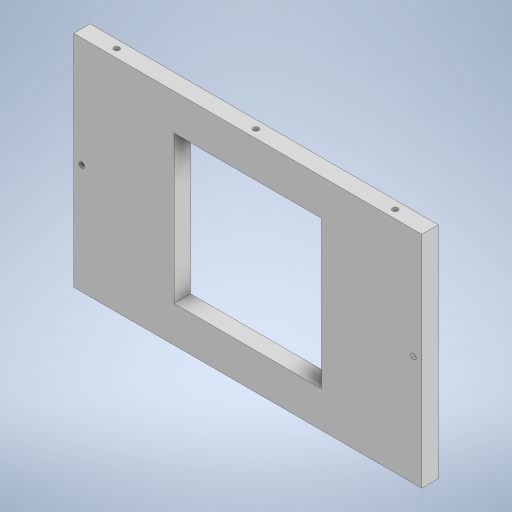
# Autodesk Inventor part: Lateral
Saved by Autodesk Inventor 2023.2 (Build 272271030, 271C)
## iProperties
Created: 2023-04-15
Part Number: Lateral
Material: Generic
Document SubType Name: Modeling
Designer: victo
Density: 1 g/cm^3
Appearance: Default
Author: victo
## iProperties of the stored document Lateral1-2_3DPrint.ipt
Created: 2023-05-16
Part Number: Lateral1-2_3DPrint
Material: Generic
Document SubType Name: Modeling
Designer: VICTOR
Density: 1 g/cm^3
Appearance: Default
Author: VICTOR
Autodesk Inventor part; units mm, degrees
ref_plane "YZ Plane" through (0, 0, 0) normal (1, 0, 0) x (0, 1, 0)
ref_plane "XZ Plane" through (0, 0, 0) normal (0, 1, 0) x (-1, 0, 0)
ref_plane "XY Plane" through (0, 0, 0) normal (0, 0, 1) x (1, 0, 0)
sketch "Sketch1" plane through (0, 0, 0) normal (0, 0, 1) x (1, 0, 0)
  line L0 (0, 0) -> (190, 0)
  line L1 (190, 0) -> (190, 120)
  line L2 (190, 120) -> (0, 120)
  line L3 (0, 120) -> (0, 0)
  dimension "d0" = 190
  dimension "d1" = 120
  constraints: 8 end point, 2 parallel, 1 horizontal, 1 perpendicular
  measures "d0" distance of L2.end L1.end
  measures "d1" distance of L1.end L0.end
extrude "Extrusion1" add sketch "Sketch1" along normal blind 9
sketch "Sketch2" plane through (0, 0, 9) normal (0, 0, 1) x (1, 0, 0)
  line L0 (190, 0) -> (190, 120) projected
  line L1 (190, 120) -> (0, 120) projected
  line L2 (0, 120) -> (0, 0) projected
  line L3 (0, 0) -> (190, 0) projected
  line L4 (135.25, 19.75) -> (54.75, 19.75)
  line L5 (54.75, 19.75) -> (54.75, 100.25)
  line L6 (54.75, 100.25) -> (135.25, 100.25)
  line L7 (135.25, 100.25) -> (135.25, 19.75)
  line L8 (135.25, 19.75) -> (54.75, 100.25) construction
  line L9 (54.75, 19.75) -> (135.25, 100.25) construction
  point P0 (95, 60)
  dimension "d4" = 80.5
  dimension "d5" = 80.5
  constraints: 12 end point, 2 midpoint, 2 parallel, 1 horizontal, 1 perpendicular
  measures "d4" distance of L5.end L6.end
  measures "d5" distance of L4.end L5.end
extrude "Extrusion2" cut sketch "Sketch2" against normal blind 10 contours L4 L5 L6 L7
sketch "Sketch3" plane through (0, 120, 0) normal (0, 1, 0) x (1, 0, 0)
  line L0 (190, 0) -> (0, 0) projected
  line L1 (0, 0) -> (0, -9) projected
  line L2 (190, -9) -> (0, -9) projected
  line L3 (190, 0) -> (190, -9) projected
  circle A0 centre (19, -4.5) radius 1.5
  circle A1 centre (95, -4.5) radius 1.5
  circle A2 centre (171, -4.5) radius 1.5
  point P0 (0, 0)
  dimension "d8" = 3
  dimension "d9" = 3
  dimension "d10" = 3
  constraints: 3 centre point
  measures "d8" diameter of A0
  measures "d9" diameter of A1
  measures "d10" diameter of A2
extrude "Extrusion3" cut sketch "Sketch3" against normal blind 10 contours A0 | A1 | A2
sketch "Sketch4" plane through (0, 0, 0) normal (0, -1, 0) x (1, 0, 0)
  circle A0 centre (19, 4.5) radius 1.5 projected
  circle A1 centre (95, 4.5) radius 1.5 projected
  circle A2 centre (171, 4.5) radius 1.5 projected
  point P0 (0, 0)
extrude "Extrusion4" cut sketch "Sketch4" against normal blind 10
sketch "Sketch5" plane through (0, 0, 9) normal (0, 0, 1) x (1, 0, 0)
  line L0 (190, 120) -> (0, 120) projected
  line L1 (0, 0) -> (190, 0) projected
  line L2 (0, 120) -> (9, 120)
  line L3 (9, 120) -> (9, 0)
  line L4 (9, 0) -> (0, 0)
  line L5 (0, 0) -> (0, 120)
  line L6 (190, 120) -> (181, 120)
  line L7 (181, 120) -> (181, 0)
  line L8 (181, 0) -> (190, 0)
  line L9 (190, 0) -> (190, 120)
  circle A0 centre (4.5, 60) radius 1.5
  circle A1 centre (185.5, 60) radius 1.5
  dimension "d15" = 9
  dimension "d16" = 9
  dimension "d17" = 3
  dimension "d18" = 3
  constraints: 16 end point, 4 parallel, 3 point on line, 2 centre point, 2 horizontal, 2 perpendicular
  measures "d15" distance of L3.end L4.end
  measures "d16" distance of L8.end L7.end
  measures "d17" diameter of A0
  measures "d18" diameter of A1
extrude "Extrusion5" cut sketch "Sketch5" against normal blind 10 contours A0 | A1
body "Solid1"
